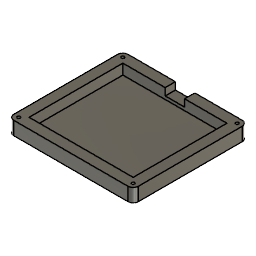
Bottom (Autodesk Fusion 360 design; units mm, degrees)
part number: 2026-03-31-19-47-08-928
Autodesk Fusion 360 part; units mm, degrees
sketch "Boceto1" plane through (0, 0, 0) normal (0, 0, 1) x (1, 0, 0)
  line L0 (50.5, -45.5) -> (-50.5, -45.5)
  line L1 (-50.5, -45.5) -> (-50.5, 45.5)
  line L2 (-50.5, 45.5) -> (50.5, 45.5)
  line L3 (50.5, 45.5) -> (50.5, -45.5)
  line L4 (50.5, -45.5) -> (-50.5, 45.5) construction
  line L5 (-50.5, -45.5) -> (50.5, 45.5) construction
  line L6 (60.5, -55.5) -> (-60.5, -55.5)
  line L7 (-60.5, -55.5) -> (-60.5, 55.5)
  line L8 (-60.5, 55.5) -> (60.5, 55.5)
  line L9 (60.5, 55.5) -> (60.5, -55.5)
  line L10 (60.5, -55.5) -> (-60.5, 55.5) construction
  line L11 (-60.5, -55.5) -> (60.5, 55.5) construction
  circle A0 centre (55.5, 50.5) radius 1.45
  circle A1 centre (55.5, -50.5) radius 1.45
  circle A2 centre (-55.5, -50.5) radius 1.45
  circle A3 centre (-55.5, 50.5) radius 1.45
  dimension "d1" = 101
  dimension "d2" = 91
  dimension "d3" = 121
  dimension "d4" = 111
  dimension "d6" = 2.9
  dimension "d10" = 2.9
  dimension "d11" = 2.9
  dimension "d12" = 2.9
  constraint horizontal L0
  constraint perpendicular L0 L1
  constraint parallel L0 L2
  constraint parallel L1 L3
  constraint coincident L4 origin
  constraint coincident L5 origin
  constraint horizontal L6
  constraint perpendicular L6 L7
  constraint parallel L6 L8
  constraint parallel L7 L9
  constraint coincident L10 origin
  constraint coincident L11 origin
  measures "d1" distance of L1.end L2.end
  measures "d2" distance of L0.end L1.end
  measures "d3" distance of L7.end L8.end
  measures "d4" distance of L6.end L7.end
  measures "d6" diameter of A0
  measures "d10" diameter of A1
  measures "d11" diameter of A2
  measures "d12" diameter of A3
extrude "Extruir1" add sketch "Boceto1" along normal blind 3 contours L0 L1 L2 L3
extrude "Extruir2" add sketch "Boceto1" along normal blind 13
sketch "Boceto2" plane through (0, 0, 13) normal (0, 0, 1) x (-1, 0, 0)
  circle A0 centre (55.5, 50.5) radius 1.45
  line L0 (50.5, -45.5) -> (-50.5, -45.5)
  line L1 (-50.5, -45.5) -> (-50.5, 45.5)
  line L2 (-50.5, 45.5) -> (50.5, 45.5)
  line L3 (50.5, 45.5) -> (50.5, -45.5)
  circle A1 centre (55.5, -50.5) radius 1.45
  circle A2 centre (-55.5, -50.5) radius 1.45
  circle A3 centre (-55.5, 50.5) radius 1.45
  line L4 (-60.5, -55.5) -> (60.5, -55.5)
  line L5 (60.5, -55.5) -> (60.5, 55.5)
  line L6 (60.5, 55.5) -> (-60.5, 55.5)
  line L7 (-60.5, 55.5) -> (-60.5, -55.5)
  line L8 (50.5, -45.5) -> (9.404, -45.5)
  line L9 (9.404, -45.5) -> (9.404, -55.5)
  line L10 (9.404, -55.5) -> (50.5, -55.5)
  line L11 (50.5, -55.5) -> (50.5, -45.5)
  line L12 (9.404, -55.5) -> (-9.396, -55.5)
  line L13 (-9.396, -55.5) -> (-9.396, -45.5)
  line L14 (-9.396, -45.5) -> (9.404, -45.5)
  line L15 (9.404, -45.5) -> (9.404, -55.5)
  line L16 (-9.396, -55.5) -> (-50.5, -55.5)
  line L17 (-50.5, -55.5) -> (-50.5, -45.5)
  line L18 (-50.5, -45.5) -> (-9.396, -45.5)
  line L19 (-9.396, -45.5) -> (-9.396, -55.5)
  dimension "d17" = 41.096
  dimension "d18" = 18.8
  constraint horizontal L8
  constraint vertical L9
  constraint horizontal L10
  constraint vertical L11
  constraint coincident L0.start L3.end
  constraint horizontal L12
  constraint vertical L13
  constraint horizontal L14
  constraint vertical L15
  constraint horizontal L16
  constraint vertical L17
  constraint horizontal L18
  constraint vertical L19
  constraint coincident L0.end L1.start
  measures "d17" distance of L0.start L8.end
  measures "d18" distance of L9.end L12.end
extrude "Extruir3" cut sketch "Boceto2" against normal blind 7 contours L0 L4 L9 L12 L13 L14 L15 L19
fillet "Empalme1" radius 5 4 edges at (60.5, 55.5, 6.5) (60.5, -55.5, 6.5) (-60.5, -55.5, 6.5) (-60.5, 55.5, 6.5)
sketch "Boceto3" plane through (0, 0, 0) normal (0, 0, 1) x (1, 0, 0)
  line L0 (29.725, -4.2847) -> (-29.5911, -4.2847) construction
  line L1 (-29.5911, -4.2847) -> (-29.5911, 6.6948) construction
  line L2 (-29.5911, 6.6948) -> (29.725, 6.6948) construction
  line L3 (29.725, 6.6948) -> (29.725, -4.2847) construction
  dimension "d23" = 15
  text T0 "NeowPad" font "Arial" height 15 bold align centre middle in box 59.3161 x 10.9795 at (29.725, -4.2847) x (-1, 0) y (0, 1) spacing 1
extrude "Extruir4" cut sketch "Boceto3" along normal blind 1 text T0
equation "d1 = 100 mm + 1 mm"
equation "d2 = 90 mm + 1 mm"
equation "d3 = 100 mm + 1 mm + 20 mm"
equation "d4 = 90 mm + 1 mm + 20 mm"
equation "d18 = 17.8 mm + 1 mm"
equation "d24 = 'NeowPad'"
